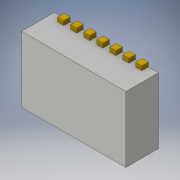
# Autodesk Inventor part: MC_BK377
Saved by Autodesk Inventor 2016 (Build 200138000, 138)
## iProperties
Created: 2016-08-30
Part Number: MC_BK377
Material: Generic
Document SubType Name: Modeling
Designer: jfixelle
Density: 1 g/cm^3
Appearance: Default
Author: jfixelle
Autodesk Inventor part; units mm, degrees
ref_plane "YZ Plane" through (0, 0, 0) normal (1, 0, 0) x (0, 1, 0)
ref_plane "XZ Plane" through (0, 0, 0) normal (0, 1, 0) x (-1, 0, 0)
ref_plane "XY Plane" through (0, 0, 0) normal (0, 0, 1) x (1, 0, 0)
sketch "Sketch1" plane through (0, 0, 0) normal (0, 0, 1) x (1, 0, 0)
  line L0 (-10.16, 6.415) -> (10.16, 6.415)
  line L1 (10.16, 6.415) -> (10.16, -6.415)
  line L2 (10.16, -6.415) -> (-10.16, -6.415)
  line L3 (-10.16, -6.415) -> (-10.16, 6.415)
  point P0 (0, 0)
  dimension "d0" = 20.32
  dimension "d1" = 10.16
  dimension "d2" = 12.83
  dimension "d3" = 6.415
  constraints: 8 end point, 2 parallel, 1 horizontal, 1 perpendicular
  measures "d0" distance of L0.start L0.end
  measures "d1" distance from line of point (0, 0) L1
  measures "d2" distance of L0.end L1.end
  measures "d3" distance from line of point (0, 0) L0
extrude "Extrusion1" add sketch "Sketch1" along normal blind 6.35
sketch "Sketch2" plane through (0, 0, 0) normal (0, 0, -1) x (-1, 0, 0)
  line L0 (8.215, 7.24) -> (7.025, 7.24)
  line L1 (7.025, 7.24) -> (7.025, 5.59)
  line L2 (7.025, 5.59) -> (8.215, 5.59)
  line L3 (8.215, 5.59) -> (8.215, 7.24)
  line L4 (10.16, 6.415) -> (-10.16, 6.415) projected
  line L5 (10.16, -6.415) -> (10.16, 6.415) projected
  point P0 (0, 0)
  dimension "d6" = 1.65
  dimension "d7" = 0.825
  dimension "d8" = 1.19
  dimension "d9" = 1.945
  constraints: 8 end point, 2 parallel, 1 horizontal, 1 perpendicular
  measures "d6" distance of L0.end L1.end
  measures "d7" distance between parallel lines of L0 L4
  measures "d8" distance of L0.start L0.end
  measures "d9" distance between parallel lines of L3 L5
extrude "Extrusion2" add sketch "Sketch2" against normal blind 1.27
pattern_linear "Rectangular Pattern1" count 7 spacing 2.54 along (1, 0, 0) of "Extrusion2"
mirror "Mirror1" about plane through (0, 0, 0) normal (0, 1, 0) of "Extrusion2", "Rectangular Pattern1"
body "Solid1"
